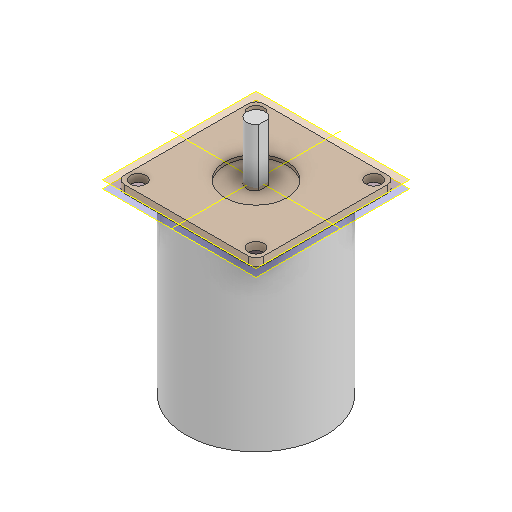
# Autodesk Inventor part: 모터
Saved by Autodesk Inventor 2027 (Build 310192000, 192)
## iProperties
Created: 2026-09-17
Part Number: 모터
Material: 일반
Document SubType Name: Modeling
Designer: User
Density: 1 g/cm^3
Appearance: 기본값
Author: User
Autodesk Inventor part; units mm, degrees
ref_plane "YZ 평면_우측면도" through (0, 0, 0) normal (1, 0, 0) x (0, 1, 0)
ref_plane "XZ 평면_평면도" through (0, 0, 0) normal (0, 1, 0) x (-1, 0, 0)
ref_plane "XY 평면_정면도" through (0, 0, 0) normal (0, 0, 1) x (1, 0, 0)
sketch "스케치1" plane through (0, 0, 0) normal (0, 1, 0) x (-1, 0, 0)
  line L0 (-40, -45) -> (40, -45)
  line L1 (45, -40) -> (45, 40)
  line L2 (40, 45) -> (-40, 45)
  line L3 (-45, 40) -> (-45, -40)
  line L4 (-45, -45) -> (45, 45) construction
  line L5 (45, -45) -> (-45, 45) construction
  line L6 (-45, 45) -> (-37.9289, 37.9289) construction
  circle A0 centre (-37.9289, 37.9289) radius 5
  circle A1 centre (-37.9289, -37.9289) radius 5
  circle A2 centre (37.9289, -37.9289) radius 5
  circle A3 centre (37.9289, 37.9289) radius 5
  arc A4 (-40, 45) -> (-45, 40) centre (-40, 40) ccw
  arc A5 (-45, -40) -> (-40, -45) centre (-40, -40) ccw
  arc A6 (40, -45) -> (45, -40) centre (40, -40) ccw
  arc A7 (45, 40) -> (40, 45) centre (40, 40) ccw
  point P0 (0, 0)
  dimension "d0" = 90
  dimension "d1" = 90
  dimension "d2" = 10
  dimension "d3" = 10
  dimension "d6" = 360
  dimension "d8" = 5
  dimension "d9" = 5
  constraints: 14 end point, 9 point on line, 8 centre point, 8 point on circle, 8 tangent, 2 equal radius, 2 midpoint, 2 parallel, 1 coincident, 1 horizontal, 1 perpendicular, 9 other
  measures "d0" distance of L5.end L4.end
  measures "d1" distance of L4.end L5.start
  measures "d2" distance of L5.end L6.end
  measures "d3" diameter of A0
  measures "d8" radius of A4
  measures "d9" radius of A5
extrude "돌출1" add sketch "스케치1" against normal blind 5
ref_plane "작업 평면1" through (0, 0, 0) normal (0, 1, 0) x (1, 0, 0)
sketch "스케치2" plane through (0, 0, 0) normal (0, 1, 0) x (1, 0, 0)
  circle A0 centre (0, 0) radius 20
  dimension "d13" = 40
  constraints: 1 centre point, 1 coincident
  measures "d13" diameter of A0
extrude "돌출3" cut sketch "스케치2" against normal blind 2
sketch "스케치3" plane through (0, 0, 0) normal (0, 1, 0) x (1, 0, 0)
  arc A0 (5, 3.3166) -> (5, -3.3166) centre (0, 0) ccw
  line L0 (0, -6) -> (0, 6) construction
  line L1 (5, -3.3166) -> (5, 3.3166)
  dimension "d14" = 12
  dimension "d15" = 5
  constraints: 4 end point, 3 point on circle, 1 centre point, 1 coincident, 1 midpoint, 1 parallel, 1 vertical
  measures "d14" diameter of A0
  measures "d15" distance between parallel lines of L0 L1
extrude "돌출2" add sketch "스케치3" along normal blind 35 and the other way blind 2
ref_plane "작업 평면2" through (0, -5, 0) normal (0, -1, 0) x (1, 0, 0)
sketch "스케치4" plane through (0, -5, 0) normal (0, -1, 0) x (1, 0, 0)
  circle A0 centre (0, 0) radius 45
  dimension "d23" = 90
  constraints: 1 centre point, 1 coincident
  measures "d23" diameter of A0
extrude "돌출4" add sketch "스케치4" along normal blind 115
